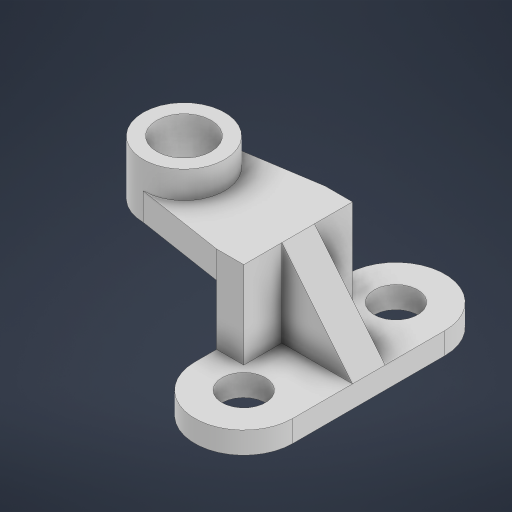
# Autodesk Inventor part: Part3
Saved by Autodesk Inventor 2024 (Build 280153000, 153)
## iProperties
Created: 2024-02-24
Part Number: Part3
Material: Generic
Document SubType Name: Modeling
Designer: Papryk
Density: 1 g/cm^3
Appearance: Default
Author: Papryk
Autodesk Inventor part; units mm, degrees
ref_plane "YZ Plane" through (0, 0, 0) normal (1, 0, 0) x (0, 1, 0)
ref_plane "XZ Plane" through (0, 0, 0) normal (0, 1, 0) x (-1, 0, 0)
ref_plane "XY Plane" through (0, 0, 0) normal (0, 0, 1) x (1, 0, 0)
sketch "Sketch1" plane through (0, 0, 0) normal (0, 1, 0) x (-1, 0, 0)
  line L0 (0, 0) -> (36, 0)
  line L1 (36, 0) -> (36, 28)
  line L2 (0, 28) -> (0, 0)
  arc A0 (36, 28) -> (0, 28) centre (18, 28) ccw
  circle A1 centre (18, 28) radius 8
  dimension "d0" = 36
  dimension "d1" = 28
  dimension "d2" = 16
  constraints: 6 end point, 2 centre point, 2 point on circle, 1 coincident, 1 horizontal, 1 parallel, 1 perpendicular
  measures "d0" distance of L2.start L1.end
  measures "d1" distance of L1.end L0.end
  measures "d2" diameter of A1
extrude "Extrusion1" add sketch "Sketch1" along normal blind 8
sketch "Sketch2" plane through (0, 0, 0) normal (0, 0, -1) x (-1, 0, 0)
  line L0 (36, 8) -> (0, 8) projected
  line L1 (36, 8) -> (26, 8)
  line L2 (26, 8) -> (26, 40)
  line L3 (26, 40) -> (36, 40)
  line L4 (36, 40) -> (36, 8)
  line L5 (26, 40) -> (0, 8)
  point P0 (0, 0)
  dimension "d5" = 10
  dimension "d6" = 32
  constraints: 10 end point, 2 parallel, 1 horizontal, 1 perpendicular
  measures "d5" distance of L2.end L3.end
  measures "d6" distance of L1.end L2.end
mirror "Mirror1" about plane through (0, 0, 0) normal (0, 0, 1) of "Extrusion1"
extrude "Extrusion2" add sketch "Sketch2" along normal mid plane 12 contours L0 L5 L2
extrude "Extrusion3" add sketch "Sketch2" along normal mid plane 40 contours L0 L2 L3 L4
sketch "Sketch3" plane through (-36, 40, -20) normal (0, 1, 0) x (1, 0, 0)
  line L0 (0, 8) -> (0, -48) projected
  circle A0 centre (-32, -20) radius 10
  circle A1 centre (-32, -20) radius 15
  line L1 (0, -48) -> (0, -40) projected
  line L2 (0, -40) -> (-32, -35)
  line L3 (0, 0) -> (10, 0) projected
  line L4 (0, 0) -> (-32, -5)
  point P0 (36, -20)
  dimension "d12" = 20
  dimension "d13" = 30
  constraints: 4 end point, 2 centre point, 2 point on circle, 1 coincident
  measures "d12" diameter of A0
  measures "d13" diameter of A1
extrude "Extrusion4" add sketch "Sketch3" against normal blind 10 contours L0 L2 A1 L4
extrude "Extrusion5" add sketch "Sketch3" along normal blind 10 and the other way blind 10 contours A1
body "Solid1"
